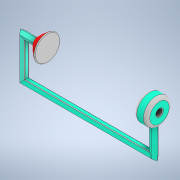
# Autodesk Inventor part: Base
Saved by Autodesk Inventor 2021 (Build 250183000, 183)
## iProperties
Created: 2021-07-29
Part Number: Base
Material: Generic
Document SubType Name: Modeling
Designer: Shammy Haider
Density: 1 g/cm^3
Appearance: Default
Author: Shammy Haider
Autodesk Inventor part; units mm, degrees
ref_plane "YZ Plane" through (0, 0, 0) normal (1, 0, 0) x (0, 1, 0)
sketch "Sketch1" plane through (0, 0, 0) normal (0, 0, 1) x (1, 0, 0)
  line L0 (-80, 60) -> (-100, 60)
  line L1 (-100, 60) -> (-100, 0)
  line L2 (-100, 0) -> (100, 0)
  line L3 (100, 0) -> (100, 45)
  point P0 (0, 0)
  dimension "d0" = 60
  dimension "d1" = 200
  dimension "d2" = 45
  dimension "d3" = 20
  dimension "d4" = 100
  dimension "d5" = 0
  constraints: 8 end point, 3 perpendicular, 1 horizontal
  measures "d0" distance of L0.end L1.end
  measures "d1" distance of L1.end L2.end
  measures "d2" distance of L2.end L3.end
  measures "d3" distance of L0.start L0.end
  measures "d4" distance from line of point (0, 0) L1
  measures "d5" distance from line of point (0, 0) L2
ref_plane "Work Plane1" through (-80, 60, 0) normal (-1, 0, 0) x (0, -1, 0)
sketch "Sketch2" plane through (-80, 60, 0) normal (-1, 0, 0) x (0, -1, 0)
  line L0 (3.6214, -3.1856) -> (-2.3057, -4.9439)
  line L1 (-2.3057, -4.9439) -> (-5.8094, 0.1498)
  line L2 (-5.8094, 0.1498) -> (-2.0478, 5.0561)
  line L3 (-2.0478, 5.0561) -> (3.7808, 2.9947)
  line L4 (3.7808, 2.9947) -> (3.6214, -3.1856)
  point P0 (60, 0)
  point P1 (-0.5521, 0.0142)
  dimension "d6" = 10
  constraints: 10 end point, 11 other
  measures "d6" vertical distance of L0.end L2.end
sweep "Sweep1" add profiles "Sketch2" path "Sketch1"
sketch "Sketch3" plane through (0, 0, 0) normal (0, 0, 1) x (1, 0, 0)
  line L0 (-80, 65.8094) -> (-105.8094, 65.8094) projected
  line L1 (-80, 65.8094) -> (-80, 70.8094)
  line L2 (-80, 70.8094) -> (-75, 70.8094)
  line L3 (-75, 70.8094) -> (-75, 75.8094)
  line L4 (-75, 75.8094) -> (-69, 75.8094)
  line L5 (-69, 75.8094) -> (-69, 80.8094)
  line L6 (-69, 80.8094) -> (-64, 80.8094)
  line L7 (-64, 80.8094) -> (-64, 60.8094)
  line L8 (-64, 60.8094) -> (-80, 60.8094)
  line L9 (-80, 56.2192) -> (-80, 62.0478) projected
  line L10 (-80, 62.0478) -> (-80, 65.8094) projected
  line L11 (-80, 65.8094) -> (-80, 60.8094)
  point P0 (0, 0)
  dimension "d9" = 20
  dimension "d10" = 15
  dimension "d11" = 10
  dimension "d12" = 5
  dimension "d13" = 6
  dimension "d14" = 5
  dimension "d15" = 5
  constraints: 18 end point, 8 perpendicular, 1 point on line, 1 vertical
  measures "d9" distance of L6.end L7.end
  measures "d10" distance between parallel lines of L8 L4
  measures "d11" distance between parallel lines of L8 L2
  measures "d12" distance between parallel lines of L7 L5
  measures "d13" distance between parallel lines of L5 L3
  measures "d14" distance between parallel lines of L3 L1
  measures "d15" distance between parallel lines of L0 L8
revolve "Revolution1" add sketch "Sketch3" angle 360 about axis through (-64, 60.8094, 0) along (-1, 0, 0)
fillet "Fillet1" radius 5 3 edges at (-80, 50.8094, 0) (-75, 45.8094, 0) (-69, 40.8094, 0)
ref_plane "Work Plane2" through (99.3421, 45, -4.0647) normal (1, 0, 0) x (0, 0, -1)
sketch "Sketch4" plane through (99.3421, 45, -4.0647) normal (1, 0, 0) x (0, 0, -1)
  circle A0 centre (-4.0647, 15.8094) radius 20 projected
  point P0 (-4.0647, -45)
extrude "Extrusion1" add sketch "Sketch4" along normal mid plane 20
sketch "Sketch5" plane through (109.3421, 60.8094, 0) normal (1, 0, 0) x (0, 0, -1)
  circle A0 centre (0, 0) radius 5
  point P0 (0, -60.8094)
  dimension "d20" = 10
  constraints: 1 centre point
  measures "d20" diameter of A0
extrude "Extrusion2" cut sketch "Sketch5" against normal blind 20
thread "Thread1"
fillet "Fillet2" radius 5 2 edges at (89.3421, 60.8094, 20) (109.3421, 60.8094, 20)
fillet "Fillet3" radius 1 11 edges at (109.3421, 60.8094, 5) (89.3421, 60.8094, 5) (96.2192, 22.4079, 2.9947) (-64, 40.8094, 0) (96.3786, 22.3431, -3.1856) (0, 3.7808, 2.9947) (0, 3.6214, -3.1856) (-96.2192, 30, 2.9947) (-96.3786, 30, -3.1856) (-88.098, 56.2192, 2.9947) (-88.1788, 56.3786, -3.1856)
body "Solid1"
